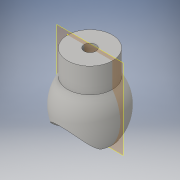
# Autodesk Inventor part: caster holder jeffreys
Saved by Autodesk Inventor 2016 (Build 200138000, 138)
## iProperties
Created: 2016-10-20
Part Number: caster holder jeffreys
Material: Generic
Document SubType Name: Modeling
Designer: pascaj
Density: 1 g/cm^3
Appearance: Default
Author: pascaj
Autodesk Inventor part; units mm, degrees
ref_plane "YZ Plane" through (0, 0, 0) normal (1, 0, 0) x (0, 1, 0)
ref_plane "XZ Plane" through (0, 0, 0) normal (0, 1, 0) x (-1, 0, 0)
sketch "Sketch1" plane through (0, 0, 0) normal (0, 0, 1) x (1, 0, 0)
  line L0 (0, 0) -> (11.43, 0)
  line L1 (11.43, 0) -> (11.43, -12.7)
  line L2 (11.43, -12.7) -> (0, -12.7)
  line L3 (0, -12.7) -> (0, 0)
  line L4 (11.43, 0) -> (11.43, -54.8894) construction
  arc A0 (0, -12.7) -> (0, -37.2615) centre (16.7117, -24.9808) ccw
  arc A1 (0, -12.7) -> (0, -37.2615) centre (33.6789, -24.9808) ccw
  dimension "d2" = 16.9672
  dimension "d3" = 12.7
  dimension "d16" = 11.43
  dimension "d17" = 54.8894
  constraints: 10 end point, 4 point on circle, 2 centre point, 2 parallel, 1 horizontal, 1 perpendicular, 1 point on line
  measures "d2" distance of A1.centre A0.centre
  measures "d3" distance between parallel lines of L2 L0
  measures "d16" distance of L0.start L0.end
  measures "d17" distance of L0.end L4.end
revolve "Revolution1" add sketch "Sketch1" angle 360 about axis through (11.43, 0, 0) along (0, -1, 0)
sketch "Sketch2" plane through (0, 0, 0) normal (0, 0, 1) x (1, 0, 0)
  line L0 (22.86, 0) -> (0, 0) projected
  line L1 (11.43, 0) -> (8.4328, 0)
  line L2 (11.43, 0) -> (11.43, -6.35)
  line L3 (11.43, -6.35) -> (8.5598, -6.35)
  line L4 (8.5598, -6.35) -> (8.5598, -4.699)
  line L5 (8.5598, -4.699) -> (8.4328, 0)
  dimension "d7" = 2.9972
  dimension "d8" = 6.35
  dimension "d9" = 2.8702
  dimension "d12" = 1.651
  constraints: 10 end point, 1 horizontal, 1 midpoint, 1 perpendicular, 1 point on line, 1 vertical
  measures "d7" distance of L1.start L1.end
  measures "d8" distance of L1.start L2.end
  measures "d9" distance of L2.end L3.end
  measures "d12" distance of L3.end L4.end
revolve "Revolution2" cut sketch "Sketch2" angle 360 about axis through (11.43, 0, 0) along (0, -1, 0)
sketch "Sketch3" plane through (0, 0, 0) normal (0, 0, 1) x (1, 0, 0)
  line L0 (22.86, -37.2615) -> (0, -37.2615) projected
  circle A0 centre (11.43, -37.2615) radius 10.3649
  point P0 (0, 0)
  constraints: 1 centre point, 1 midpoint
extrude "Extrusion1" cut sketch "Sketch3" along normal mid plane 635
sketch "Sketch4" plane through (0, 0, 0) normal (0, 0, 1) x (1, 0, 0)
  point P0 (0, 0)
sketch "Sketch5" plane through (11.43, 0, 0) normal (0, 1, 0) x (1, 0, 0)
  point P0 (-11.43, 0)
body "Solid1"
